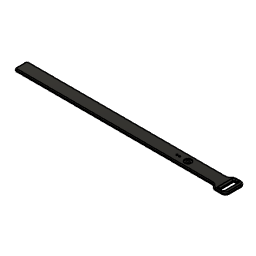
Bias Band Fusion File (Autodesk Fusion 360 design; units mm, degrees)
Autodesk Fusion 360 part; units mm, degrees
note: some values were not read from the file. Chosen so that the rebuilt part matches the saved one: which face or edge a step refers to; which pieces of a blend or face edit are solid.
sketch "Sketch1" plane through (0, 0, 0) normal (0, 0, 1) x (1, 0, 0)
  line L0 (125, 7.5) -> (-125, 7.5)
  line L1 (-125, 7.5) -> (-125, -7.5)
  line L2 (-125, -7.5) -> (125, -7.5)
  line L3 (125, -7.5) -> (125, 7.5)
  line L4 (125, 7.5) -> (-125, -7.5) construction
  line L5 (-125, 7.5) -> (125, -7.5) construction
  line L6 (80, 7.5) -> (80, 11.5)
  line L7 (80, 11.5) -> (125, 11.5)
  line L8 (125, 11.5) -> (125, 7.5)
  line L9 (1.75, 0) -> (22.5, 0)
  line L10 (125, -11.5) -> (125, -7.5)
  line L11 (80, -11.5) -> (125, -11.5)
  line L12 (80, -7.5) -> (80, -11.5)
  line L13 (95, 11.5) -> (95, -11.5)
  line L14 (110, 11.5) -> (110, -11.5)
  dimension "d1" = 250
  dimension "d2" = 15
  dimension "d7" = 4
  dimension "d8" = 45
  dimension "d9" = 15
  dimension "d10" = 15
  constraint horizontal L0
  constraint perpendicular L0 L1
  constraint parallel L0 L2
  constraint parallel L1 L3
  constraint coincident L4 origin
  constraint coincident L5 origin
  constraint coincident L0 L6.start
  constraint perpendicular L0 L6
  constraint perpendicular L6 L7
  constraint perpendicular L0 L8
  constraint symmetric L0.start L9 L2.end
  constraint symmetric L6.start L9 L12.start
  constraint symmetric L6.end L9 L11.start
  constraint symmetric L7.end L9 L10.start
  constraint coincident L7 L13.start
  constraint coincident L11 L13.end
  constraint perpendicular L11 L13
  constraint coincident L7 L14.start
  constraint coincident L11 L14.end
  constraint perpendicular L11 L14
  measures "d1" distance of L1.end L2.end
  measures "d2" distance of L0.end L1.end
  measures "d7" distance of L6.start L6.end
  measures "d8" distance of L6.end L7.end
  measures "d9" distance of L13 L14
  measures "d10" distance of L8 L14
extrude "Extrude1" add sketch "Sketch1" along normal blind 3 contours L0 L1 L2 L13 | L0 L2 L13 L14 | L0 L7 L8 L14 | L0 L2 L3 L14 | L2 L10 L11 L14
fillet "Fillet2" radius 5 6 edges at (110, 11.5, 1.5) (110, 7.5, 1.5) (125, 11.5, 1.5) (110, -11.5, 1.5) (125, -11.5, 1.5) (110, -7.5, 1.5)
sketch "Sketch2" plane through (0, 0, 3) normal (0, 0, 1) x (-1, 0, 0)
  line L0 (-106.899, -7.5) -> (125, -7.5)
  line L1 (125, -7.5) -> (125, 7.5)
  line L2 (125, 7.5) -> (-105.101, 7.5)
  line L3 (-117.4495, -11.5) -> (-116.5505, 11.5) construction
  line L4 (-119.5, -8.75) -> (-114.5, -8.75)
  line L5 (-114.5, -8.75) -> (-114.5, 8.75)
  line L6 (-114.5, 8.75) -> (-119.5, 8.75)
  line L7 (-119.5, 8.75) -> (-119.5, -8.75)
  line L8 (-119.5, -8.75) -> (-114.5, 8.75) construction
  line L9 (-114.5, -8.75) -> (-119.5, 8.75) construction
  arc A0 (-109.101, 9.5) -> (-113.101, 11.5) centre (-113.101, 6.5) ccw
  line L10 (-113.101, 11.5) -> (-120, 11.5)
  arc A1 (-120, 11.5) -> (-125, 6.5) centre (-120, 6.5) ccw
  line L11 (-120, -11.5) -> (-114.899, -11.5)
  arc A2 (-114.899, -11.5) -> (-110.899, -9.5) centre (-114.899, -6.5) ccw
  arc A3 (-106.899, -7.5) -> (-110.899, -9.5) centre (-106.899, -12.5) ccw
  arc A4 (-109.101, 9.5) -> (-105.101, 7.5) centre (-105.101, 12.5) ccw
  line L12 (-125, 6.5) -> (-125, -6.5)
  arc A5 (-125, -6.5) -> (-120, -11.5) centre (-120, -6.5) ccw
  point P0 (-62.5, 0)
  point P1 (-117, 0)
  dimension "d15" = 5
  dimension "d16" = 17.5
  constraint horizontal L4
  constraint perpendicular L4 L5
  constraint parallel L4 L6
  constraint parallel L5 L7
  constraint coincident L8 P1
  constraint coincident L9 P1
  constraint midpoint L3 P1
  constraint midpoint L3.start L11
  constraint midpoint L3.end L10
  measures "d15" distance of L5.end L6.end
  measures "d16" distance of L4.end L5.end
extrude "Extrude2" cut sketch "Sketch2" against normal through all contours L4 L5 L6 L7
fillet "Fillet3" radius 1 4 edges at (114.5, -8.75, 1.5) (114.5, 8.75, 1.5) (119.5, 8.75, 1.5) (119.5, -8.75, 1.5)
fillet "Fillet5" radius 2.5 2 edges at (-125, -7.5, 1.5) (-125, 7.5, 1.5)
fillet "Fillet4" radius 1 14 faces at (125, -2.1667, 1) (123.9303, -9.5908, 2) (115.4007, -11.5, 1) (109.2373, -9.6736, 2) (105.3217, -7.5049, 1) (29.234, -7.5, 2) (-123.4292, -7.3209, 1) (-125, 1.6667, 1) (-123.4292, 7.3209, 1) (30.4327, 7.5, 1) (110.3096, 8.8438, 2) (111.6531, 10.3032, 2) (116.5993, 11.5, 1) (124.9774, 6.9753, 2)
chamfer "Chamfer1" distance 1.5 angle 45 8 edges at (114.5, 0, 3) (114.7929, 8.4571, 3) (117, 8.75, 3) (119.2071, 8.4571, 3) (119.5, 0, 3) (119.2071, -8.4571, 3) (117, -8.75, 3) (114.7929, -8.4571, 3)
sketch "Sketch5" plane through (0, 0, 3) normal (0, 0, 1) x (-1, 0, 0)
  line L0 (-124, 6.5) -> (-124, -6.5)
  arc A0 (-124, -6.5) -> (-120, -10.5) centre (-120, -6.5) ccw
  line L1 (-120, -10.5) -> (-114.899, -10.5)
  arc A1 (-114.899, -10.5) -> (-111.699, -8.9) centre (-114.899, -6.5) ccw
  arc A2 (-106.899, -6.5) -> (-111.699, -8.9) centre (-106.899, -12.5) ccw
  line L2 (-106.899, -6.5) -> (122.5, -6.5)
  arc A3 (122.5, -6.5) -> (124, -5) centre (122.5, -5) ccw
  line L3 (124, -5) -> (124, 5)
  arc A4 (124, 5) -> (122.5, 6.5) centre (122.5, 5) ccw
  line L4 (122.5, 6.5) -> (-105.101, 6.5)
  arc A5 (-109.901, 8.9) -> (-105.101, 6.5) centre (-105.101, 12.5) ccw
  arc A6 (-109.901, 8.9) -> (-113.101, 10.5) centre (-113.101, 6.5) ccw
  line L5 (-113.101, 10.5) -> (-120, 10.5)
  arc A7 (-120, 10.5) -> (-124, 6.5) centre (-120, 6.5) ccw
  line L6 (-113, 7.75) -> (-113, -7.75)
  arc A8 (-115.5, -10.25) -> (-113, -7.75) centre (-115.5, -7.75) ccw
  line L7 (-115.5, -10.25) -> (-118.5, -10.25)
  arc A9 (-121, -7.75) -> (-118.5, -10.25) centre (-118.5, -7.75) ccw
  line L8 (-121, -7.75) -> (-121, 7.75)
  arc A10 (-118.5, 10.25) -> (-121, 7.75) centre (-118.5, 7.75) ccw
  line L9 (-118.5, 10.25) -> (-115.5, 10.25)
  arc A11 (-113, 7.75) -> (-115.5, 10.25) centre (-115.5, 7.75) ccw
  circle A12 centre (-70, 0) radius 3.95
  dimension "d37" = 7.9
  dimension "d43" = 70
  constraint horizontal origin A12.centre
  measures "d37" diameter of A12
  measures "d43" horizontal distance of origin A12.centre
extrude "Extrude5" cut sketch "Sketch5" against normal blind 1 contours A12
sketch "Sketch6" plane through (0, 0, 2) normal (0, 0, 1) x (-1, 0, 0)
  circle A0 centre (-70, 0) radius 3.95
  circle A1 centre (-70, 0) radius 2
  dimension "d40" = 4
  constraint concentric A0 A1
  measures "d40" diameter of A1
extrude "Extrude6" cut sketch "Sketch6" against normal through all contours A1
sketch "Sketch7" plane through (0, 0, 3) normal (0, 0, 1) x (-1, 0, 0)
  circle A0 centre (-70, 0) radius 3.95
  line L0 (-124, 6.5) -> (-124, -6.5)
  arc A1 (-124, -6.5) -> (-120, -10.5) centre (-120, -6.5) ccw
  line L1 (-120, -10.5) -> (-114.899, -10.5)
  arc A2 (-114.899, -10.5) -> (-111.699, -8.9) centre (-114.899, -6.5) ccw
  arc A3 (-106.899, -6.5) -> (-111.699, -8.9) centre (-106.899, -12.5) ccw
  line L2 (-106.899, -6.5) -> (122.5, -6.5)
  arc A4 (122.5, -6.5) -> (124, -5) centre (122.5, -5) ccw
  line L3 (124, -5) -> (124, 5)
  arc A5 (124, 5) -> (122.5, 6.5) centre (122.5, 5) ccw
  line L4 (122.5, 6.5) -> (-105.101, 6.5)
  arc A6 (-109.901, 8.9) -> (-105.101, 6.5) centre (-105.101, 12.5) ccw
  arc A7 (-109.901, 8.9) -> (-113.101, 10.5) centre (-113.101, 6.5) ccw
  line L5 (-113.101, 10.5) -> (-120, 10.5)
  arc A8 (-120, 10.5) -> (-124, 6.5) centre (-120, 6.5) ccw
  line L6 (-113, 7.75) -> (-113, -7.75)
  arc A9 (-115.5, -10.25) -> (-113, -7.75) centre (-115.5, -7.75) ccw
  line L7 (-115.5, -10.25) -> (-118.5, -10.25)
  arc A10 (-121, -7.75) -> (-118.5, -10.25) centre (-118.5, -7.75) ccw
  line L8 (-121, -7.75) -> (-121, 7.75)
  arc A11 (-118.5, 10.25) -> (-121, 7.75) centre (-118.5, 7.75) ccw
  line L9 (-118.5, 10.25) -> (-115.5, 10.25)
  arc A12 (-113, 7.75) -> (-115.5, 10.25) centre (-115.5, 7.75) ccw
  circle A13 centre (-60, 0) radius 1
  circle A14 centre (-57, 0) radius 1
  dimension "d44" = 2
  dimension "d45" = 10
  dimension "d48" = 3
  constraint horizontal A0.centre A13.centre
  constraint equal A13 A14
  constraint horizontal A13.centre A14.centre
  measures "d44" diameter of A13
  measures "d45" horizontal distance of A0.centre A13.centre
  measures "d48" distance of A13.centre A14.centre
extrude "Extrude7" cut sketch "Sketch7" along normal through all and the other way through all contours A13 | A14
